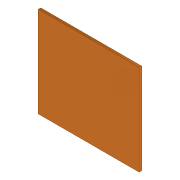
# Autodesk Inventor part: side_wall
Saved by Autodesk Inventor 2020 (Build 240168000, 168)
## iProperties
Created: 2021-05-08
Part Number: side_wall
Material: Gold
Document SubType Name: Modeling
Designer: Hsu Daniel
Density: 19.3 g/cm^3
Appearance: Metal 1600F Hot
Author: Hsu Daniel
Autodesk Inventor part; units mm, degrees
ref_plane "YZ Plane" through (0, 0, 0) normal (1, 0, 0) x (0, 1, 0)
ref_plane "XZ Plane" through (0, 0, 0) normal (0, 1, 0) x (-1, 0, 0)
ref_plane "XY Plane" through (0, 0, 0) normal (0, 0, 1) x (1, 0, 0)
sketch "Sketch1" plane through (0, 0, 0) normal (0, 0, 1) x (1, 0, 0)
  line L0 (0, 0) -> (132.6, 0)
  line L1 (132.6, 0) -> (132.6, 200)
  line L2 (132.6, 200) -> (0, 200)
  line L3 (0, 200) -> (0, 0)
  dimension "d0" = 200
  dimension "d1" = 132.6
  constraints: 8 end point, 2 parallel, 1 horizontal, 1 perpendicular
  measures "d0" distance of L0.end L1.end
  measures "d1" distance of L1.end L2.end
extrude "Extrusion1" add sketch "Sketch1" along normal blind 5.5
sketch "Sketch3" plane through (0, 0, 5.5) normal (0, 0, 1) x (1, 0, 0)
  line L0 (0, 200) -> (-90, 200)
  line L1 (-90, 200) -> (-90, 0)
  line L2 (-90, 0) -> (0, 0)
  line L3 (0, 0) -> (0, 200)
  line L4 (0, 0) -> (132.6, 0) projected
  point P0 (132.6, 200)
  dimension "d8" = 90
  constraints: 8 end point, 2 parallel, 1 collinear, 1 horizontal, 1 perpendicular
  measures "d8" distance of L2.end L1.end
extrude "Extrusion3" add sketch "Sketch3" against normal blind 5.5
sketch "Sketch2" plane through (0, 0, 5.5) normal (0, 0, 1) x (1, 0, 0)
  line L0 (50.0404, 188.6001) -> (118.0696, 188.6001)
  line L1 (118.0696, 188.6001) -> (118.0696, 180.6348)
  line L2 (118.0696, 180.6348) -> (50.0404, 180.6348)
  line L3 (50.0404, 180.6348) -> (50.0404, 188.6001)
  point P0 (0, 0)
  constraints: 8 end point, 2 parallel, 1 horizontal, 1 perpendicular
equation "\"d0\" = sidewallheight"
equation "\"d1\" = sidewallL"
equation "\"d8\" = wireL"
equation "\"thick\" = 0.5"
equation "\"lrlr\" = 19"
equation "\"lrmid\" = 19.9"
equation "\"lrdepth\" = 3.3"
equation "\"mlr\" = 16.6"
equation "\"mmid\" = 24.7"
equation "\"mdepth\" = 4.5"
equation "\"lrltotal\" = 126.6"
equation "\"mltotal\" = 126.6"
equation "\"lrbetween\" = 52.1"
equation "\"mbetween\" = 49.5"
equation "\"toler\" = 1"
equation "\"tight\" = 0.08"
equation "\"stuckw\" = 6"
equation "\"sidewallL\" = 132.6"
equation "\"sidewallheight\" = 200"
equation "\"heaterH\" = 117.3"
equation "\"stickL\" = 3.5"
equation "\"wireH\" = 25"
equation "\"wireL\" = 90"
body "Solid1"
